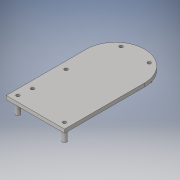
# Autodesk Inventor part: topPlate
Saved by Autodesk Inventor 2016 (Build 200138000, 138)
## iProperties
Created: 2016-03-13
Part Number: topPlate
Material: Generic
Document SubType Name: Modeling
Designer: ahenle
Density: 1 g/cm^3
Appearance: Default
Author: ahenle
Autodesk Inventor part; units mm, degrees
ref_plane "YZ Plane" through (0, 0, 0) normal (1, 0, 0) x (0, 1, 0)
ref_plane "XZ Plane" through (0, 0, 0) normal (0, 1, 0) x (-1, 0, 0)
ref_plane "XY Plane" through (0, 0, 0) normal (0, 0, 1) x (1, 0, 0)
sketch "Sketch2" plane through (0, 0, 0) normal (0, 1, 0) x (-1, 0, 0)
  line L0 (0, 0) -> (80, 0)
  line L1 (80, 0) -> (80, -110)
  line L2 (0, -110) -> (0, 0)
  arc A0 (0, -110) -> (80, -110) centre (40, -110) ccw
  dimension "d3" = 110
  dimension "d4" = 80
  dimension "d75" = 40
  constraints: 6 end point, 2 point on circle, 1 centre point, 1 horizontal, 1 parallel, 1 perpendicular
  measures "d3" distance of L0.end L1.end
  measures "d4" distance of L0.start L0.end
  measures "d75" radius of A0
extrude "Extrusion1" add sketch "Sketch2" along normal blind 5
sketch "Sketch3" plane through (0, 5, 0) normal (0, 1, 0) x (1, 0, 0)
  line L0 (-80, 0) -> (0, 0) projected
  line L1 (-80, 0) -> (-70, 0)
  line L2 (-70, 26.1273) -> (-70, 72.1273) construction
  line L3 (-80, 110) -> (-80, 0) projected
  dimension "d78" = 26.1273
  dimension "d79" = 10
  dimension "d80" = 46
  constraints: 4 end point, 1 point on line, 1 vertical
  measures "d78" distance from line of L0 L2.start
  measures "d79" distance between parallel lines of L3 L2
  measures "d80" distance of L2.start L2.end
hole "Hole1" at (-70, 5, -26.1273) at (-70, 5, -72.1273) direction (0, -1, 0) diameter 4.5 end through all clearance for "Flat Head Machine Screw" size "M4" standard "Ansi Metric M Profile"
sketch "Sketch5" plane through (0, 0, 0) normal (0, -1, 0) x (1, 0, 0)
  line L0 (-80, 0) -> (0, 0) construction
  line L1 (-80, 0) -> (-80, -6.0402) construction
  line L2 (-80, 0) -> (-80, -10) construction
  line L3 (-80, -110) -> (-80, 0) construction
  line L4 (-80, 0) -> (-80, -8) construction
  line L5 (-80, -8) -> (-72, -8) construction
  line L6 (-40, 0) -> (-40, -150) construction
  arc A0 (-80, -110) -> (0, -110) centre (-40, -110) ccw projected
  line L7 (-40, -150) -> (-40, -140) construction
  line L8 (-59.3649, -145) -> (-59.3649, -137) construction
  circle A1 centre (-72, -8) radius 3
  circle A2 centre (-8, -8) radius 3
  circle A3 centre (-59.3649, -137) radius 3
  circle A4 centre (-20.6351, -137) radius 3
  dimension "d34" = 8
  dimension "d35" = 8
  dimension "d41" = 8
  dimension "d52" = 6
  dimension "d53" = 6
  constraints: 14 end point, 4 centre point, 2 point on circle, 2 symmetric about line, 2 vertical, 1 coincident, 1 horizontal, 1 midpoint, 1 point on line, 2 other
  measures "d34" distance of L0.start L4.end
  measures "d35" distance of L4.end L5.end
  measures "d41" distance of L8.start L8.end
  measures "d52" diameter of A1
  measures "d53" diameter of A3
extrude "Extrusion2" add sketch "Sketch5" along normal blind 17
sketch "Sketch7" plane through (-8, -17, -8) normal (0, -1, 0) x (1, 0, 0)
  circle A0 centre (0, 0) radius 6.9493 construction
  circle A1 centre (-64, 0) radius 13.6969 construction
  circle A2 centre (-51.3649, -129) radius 7.4526 construction
  circle A3 centre (-12.6351, -129) radius 11.0771 construction
  circle A4 centre (0, 0) radius 3 construction
  circle A5 centre (-64, 0) radius 3 construction
  circle A6 centre (-51.3649, -129) radius 3 construction
  circle A7 centre (-12.6351, -129) radius 3 construction
  circle A8 centre (-64, 0) radius 3 construction
  circle A9 centre (-51.3649, -129) radius 3 construction
  point P0 (8, 8)
  constraints: 4 centre point, 4 coincident, 4 concentric
hole "Hole3" at (-8, -17, -8) at (-72, -17, -8) at (-59.3649, -17, -137) at (-20.6351, -17, -137) direction (0, 1, 0) diameter 4.5 end through all clearance for "Flat Head Machine Screw" size "M4" standard "Ansi Metric M Profile"
body "Solid1"
